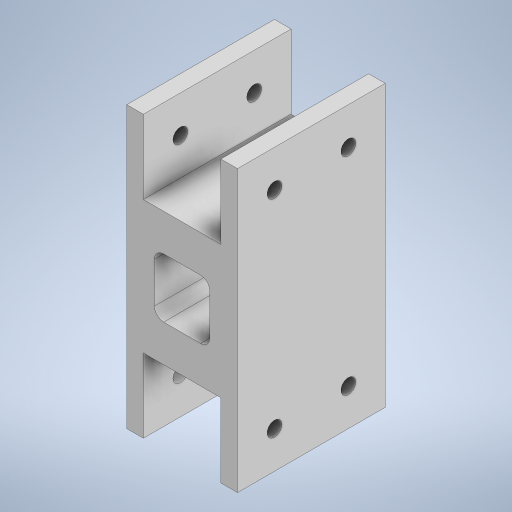
# Autodesk Inventor part: Arm_H-Bracket
Saved by Autodesk Inventor 2024 (Build 280153000, 153)
## iProperties
Created: 2025-02-18
Part Number: Arm_H-Bracket
Material: Generic
Document SubType Name: Modeling
Designer: v
Density: 1 g/cm^3
Appearance: Default
Author: v
Autodesk Inventor part; units mm, degrees
ref_plane "YZ Plane" through (0, 0, 0) normal (1, 0, 0) x (0, 1, 0)
ref_plane "XZ Plane" through (0, 0, 0) normal (0, 1, 0) x (-1, 0, 0)
ref_plane "XY Plane" through (0, 0, 0) normal (0, 0, 1) x (1, 0, 0)
sketch "Bracket-CrossArea" plane through (0, 0, 0) normal (0, 0, 1) x (1, 0, 0)
  line L0 (-20.4892, 69.1468) -> (-20.4892, -27.3732)
  line L1 (-20.4892, -27.3732) -> (-14.1392, -27.3732)
  line L2 (-14.1392, -27.3732) -> (-14.1392, -1.9732)
  line L3 (-14.1392, -1.9732) -> (11.2608, -1.9732)
  line L4 (11.2608, -1.9732) -> (11.2608, -27.3732)
  line L5 (11.2608, -27.3732) -> (17.6108, -27.3732)
  line L6 (17.6108, -27.3732) -> (17.6108, 69.1468)
  line L7 (17.6108, 69.1468) -> (11.2608, 69.1468)
  line L8 (11.2608, 69.1468) -> (11.2608, 43.7468)
  line L9 (11.2608, 43.7468) -> (-14.1392, 43.7468)
  line L10 (-14.1392, 43.7468) -> (-14.1392, 69.1468)
  line L11 (-20.4892, 69.1468) -> (-14.1392, 69.1468)
  point P0 (0, 0)
  dimension "d3" = 6.35
  dimension "d4" = 96.52
  dimension "d5" = 25.4
  dimension "d6" = 25.4
  dimension "d7" = 6.35
  dimension "d10" = 25.4
  constraints: 24 end point, 7 perpendicular, 7 point on line, 1 horizontal, 1 vertical
  measures "d3" distance of L6.end L7.end
  measures "d4" distance of L5.end L6.end
  measures "d5" distance of L7.end L8.end
  measures "d6" distance of L3.end L4.end
  measures "d7" distance of L0.start L10.end
  measures "d10" distance of L8.end L9.end
extrude "HBracket_3DShape" add sketch "Bracket-CrossArea" along normal blind 50.8
sketch "Sketch2" plane through (0, 0, 50.8) normal (0, 0, 1) x (1, 0, 0)
  line L0 (-10.9642, 31.0468) -> (8.0858, 31.0468)
  line L1 (8.0858, 31.0468) -> (8.0858, 10.7268)
  line L2 (8.0858, 10.7268) -> (-10.9642, 10.7268)
  line L3 (-10.9642, 10.7268) -> (-10.9642, 31.0468)
  line L4 (11.2608, 43.7468) -> (-14.1392, 43.7468) projected
  line L5 (-14.1392, -1.9732) -> (11.2608, -1.9732) projected
  line L6 (-14.1392, 43.7468) -> (-14.1392, 69.1468) projected
  line L7 (11.2608, 69.1468) -> (11.2608, 43.7468) projected
  line L8 (17.6108, -27.3732) -> (17.6108, 69.1468) projected
  line L9 (-20.4892, 69.1468) -> (-20.4892, -27.3732) projected
  point P0 (0, 0)
  dimension "d11" = 12.7
  dimension "d12" = 12.7
  dimension "d29" = 9.525
  dimension "d30" = 9.525
  constraints: 8 end point, 2 parallel, 1 horizontal, 1 perpendicular
  measures "d11" distance between parallel lines of L0 L4
  measures "d12" distance between parallel lines of L5 L2
  measures "d29" distance between parallel lines of L8 L1
  measures "d30" distance between parallel lines of L9 L3
extrude "MiddleHole" cut sketch "Sketch2" against normal through all
fillet "RoundedInside" radius 3.175 4 edges at (-10.9642, 10.7268, 25.4) (-10.9642, 31.0468, 25.4) (8.0858, 31.0468, 25.4) (8.0858, 10.7268, 25.4)
sketch "Sketch4" plane through (17.6108, -27.3732, 0) normal (1, 0, 0) x (0, 0, -1)
  line L0 (0, 71.12) -> (-50.8, 71.12) projected
  line L1 (0, 71.12) -> (-50.8, 71.12) projected
  line L2 (0, 0) -> (-50.8, 0) projected
  line L3 (0, 25.4) -> (-50.8, 25.4) projected
  line L4 (0, 0) -> (0, 96.52) projected
  line L5 (0, 96.52) -> (-50.8, 96.52) projected
  line L6 (-50.8, 0) -> (-50.8, 96.52) projected
  line L7 (0, 0) -> (-50.8, 0) projected
  point P0 (0, 27.3732)
  point P1 (-38.1, 83.82)
  point P2 (-12.7, 83.82)
  point P3 (-38.1, 12.7)
  point P4 (-12.7, 12.7)
  dimension "d48" = 12.7
  dimension "d49" = 12.7
  dimension "d52" = 25.4
  dimension "d55" = 71.12
  constraints: 1 horizontal, 1 vertical, 3 other
  measures "d48" distance from line of L6 point (-38.1, 83.82)
  measures "d49" distance from line of L5 point (-38.1, 83.82)
  measures "d52" distance of point (-38.1, 83.82) point (-12.7, 83.82)
  measures "d55" distance of point (-38.1, 83.82) point (-38.1, 12.7)
hole "Screw Holes" at (17.6108, 56.4468, 38.1) at (17.6108, 56.4468, 12.7) at (17.6108, -14.6732, 38.1) at (17.6108, -14.6732, 12.7) direction (-1, 0, 0) diameter 5.1054 end through all clearance for "Hex Machine Screw" size "#10" standard "Ansi Unified Screw Threads"
sketch "GapSpacing" plane through (0, 0, 50.8) normal (0, 0, 1) x (1, 0, 0)
  line L0 (-20.4892, -27.3732) -> (-14.1392, -27.3732) projected
  line L1 (-14.1392, -27.3732) -> (-14.1392, -1.9732) projected
  line L2 (-14.1392, -1.9732) -> (11.2608, -1.9732) projected
  line L3 (11.2608, -1.9732) -> (11.2608, -27.3732) projected
  line L4 (11.2608, -27.3732) -> (17.6108, -27.3732) projected
  line L5 (17.6108, -27.3732) -> (17.6108, 69.1468) projected
  line L6 (17.6108, 69.1468) -> (11.2608, 69.1468) projected
  line L7 (11.2608, 69.1468) -> (11.2608, 43.7468) projected
  line L8 (11.2608, 43.7468) -> (-14.1392, 43.7468) projected
  line L9 (-14.1392, 43.7468) -> (-14.1392, 69.1468) projected
  line L10 (-14.1392, 69.1468) -> (-20.4892, 69.1468) projected
  line L11 (-20.4892, 69.1468) -> (-20.4892, -27.3732) projected
  line L12 (-14.7742, 43.7468) -> (11.8958, 43.7468)
  line L13 (11.8958, 43.7468) -> (11.8958, 73.025)
  line L14 (11.8958, 73.025) -> (-14.7742, 73.025)
  line L15 (-14.7742, 73.025) -> (-14.7742, 43.7468)
  line L16 (-14.7742, -30.1625) -> (11.8958, -30.1625)
  line L17 (11.8958, -30.1625) -> (11.8958, -1.9732)
  line L18 (11.8958, -1.9732) -> (-14.7742, -1.9732)
  line L19 (-14.7742, -1.9732) -> (-14.7742, -30.1625)
  point P0 (-14.7742, -27.3732)
  point P1 (11.8958, -27.3732)
  point P2 (11.8958, 69.1468)
  point P3 (-14.7742, 69.1468)
  point P4 (-14.1392, 43.7468)
  point P5 (-14.1392, 43.7468)
  dimension "d58" = 0.635
  dimension "d59" = 0.635
  dimension "d62" = 0.635
  dimension "d63" = 0.635
  constraints: 16 end point, 4 parallel, 2 horizontal, 2 perpendicular
  measures "d58" distance between parallel lines of L9 L15
  measures "d59" distance between parallel lines of L7 L13
  measures "d62" distance between parallel lines of L1 L19
  measures "d63" distance between parallel lines of L3 L17
extrude "GapSpace" cut sketch "GapSpacing" against normal through all contours L19 L18 L1 L0 | L0 L1 L2 L3 L4 L17 L16 L19 | L15 L14 L13 L6 L7 L8 L9 L10 | L10 L9 L12 L15 | L18 L17 L4 L3 | L7 L6 L13 L12
equation "\"d6\" = d5"
equation "\"d7\" = d3"
equation "\"d12\" = d11"
equation "\"d30\" = d29"
equation "\"d59\" = d58"
equation "\"d62\" = d58"
equation "\"d63\" = d58"
body "Solid1"
